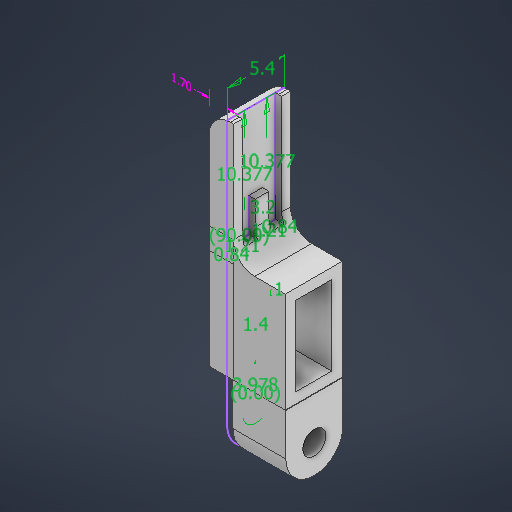
# Autodesk Inventor part: StereotaxBotHolderPartA_CH_v3
Saved by Autodesk Inventor 2026.1 (Build 301233000, 233)
## iProperties
Created: 2025-07-30
Part Number: StereotaxBotHolderPartA_CH_v3
Material: Generic
Document SubType Name: Modeling
Designer: Chris
Density: 1 g/cm^3
Appearance: Default
Author: Chris
Autodesk Inventor part; units mm, degrees
ref_plane "YZ Plane" through (0, 0, 0) normal (1, 0, 0) x (0, 1, 0)
ref_plane "XZ Plane" through (0, 0, 0) normal (0, 1, 0) x (-1, 0, 0)
ref_plane "XY Plane" through (0, 0, 0) normal (0, 0, 1) x (1, 0, 0)
sketch "Sketch1" plane through (0, 0, 0) normal (1, 0, 0) x (0, 1, 0)
  circle A0 centre (-13.4667, -0.1234) radius 1.1
  arc A1 (-13.4669, 2.577) -> (-13.4667, -2.8238) centre (-13.4667, -0.1234) ccw
  line L0 (-13.4669, 2.577) -> (-9.4882, 2.5774)
  line L1 (-9.4879, -2.8234) -> (-13.4667, -2.8238)
  line L2 (0.0118, -2.8234) -> (-9.4879, -2.8234)
  line L3 (-0.9882, -1.8234) -> (-8.4882, -1.8234)
  line L4 (-8.4882, -1.8234) -> (-8.4882, 1.5766)
  line L5 (-8.4882, 1.5766) -> (-0.9882, 1.5766)
  line L6 (-0.9882, 1.5766) -> (-0.9882, -1.8234)
  circle A2 centre (-4.7382, -0.1234) radius 1.1
  line L7 (-9.4882, 2.5774) -> (0.0115, 2.5783)
  line L8 (0.0118, -2.8234) -> (2.0118, -2.8234)
  line L9 (2.0118, 2.5766) -> (0.0115, 2.5783)
  line L10 (2.0118, 2.5766) -> (11.4892, 2.5766)
  line L11 (11.4892, -2.8234) -> (2.0118, -2.8234)
  line L12 (11.4892, -2.8234) -> (11.4892, 2.5766)
  line L13 (11.4892, 2.5766) -> (1.1118, 2.5766)
  line L14 (1.1118, 2.5766) -> (1.1118, 1.7366)
  line L15 (1.1118, 1.7366) -> (11.4892, 1.7366)
  line L16 (11.4892, 1.7366) -> (11.4892, 2.5766)
  line L17 (11.4892, -2.8234) -> (1.1118, -2.8234)
  line L18 (1.1118, -2.8234) -> (1.1118, -1.9834)
  line L19 (1.1118, -1.9834) -> (11.4892, -1.9834)
  line L20 (11.4892, -1.9834) -> (11.4892, -2.8234)
  line L21 (1.1118, -1.9834) -> (1.1118, -0.7734)
  line L22 (1.1118, 1.7366) -> (1.1118, 0.5266)
  line L23 (1.1118, 1.7366) -> (2.3218, 1.7366) construction
  line L24 (1.1118, 0.5266) -> (4.3118, 0.5266)
  line L25 (4.3118, 0.5266) -> (4.3118, -0.7734)
  line L26 (4.3118, -0.7734) -> (1.1118, -0.7734)
  line L27 (-13.4667, -0.1234) -> (-9.4882, -0.1234)
  line L28 (-13.4667, -0.1234) -> (-9.4882, -0.1234) construction
  line L29 (-9.4882, -0.1234) -> (-9.4879, -2.8234)
  line L30 (-9.4882, 2.5774) -> (-9.4882, -0.1234)
  line L31 (-9.4882, -2.8234) -> (0.0118, -2.8234)
  line L32 (0.0118, -2.8234) -> (0.0118, 2.5766)
  line L33 (0.0118, 2.5766) -> (-9.4882, 2.5766)
  line L34 (-9.4882, 2.5766) -> (-9.4882, -2.8234)
  circle A3 centre (-4.7382, -0.1234) radius 2.5
  point P0 (0, 0)
  point P1 (-9.4882, 2.5766)
  dimension "d2" = 5.4
  dimension "d3" = 10.3774
  dimension "d4" = 0.84
  dimension "d5" = 10.3774
  dimension "d6" = 0.84
  dimension "d7" = 1.21
  dimension "d8" = 1.21
  dimension "d9" = 90
  dimension "d10" = 3.2
  dimension "d11" = 3.9785
  dimension "d12" = 0
  dimension "d17" = 1
  dimension "d27" = 1.4
  constraints: 70 end point, 6 horizontal, 5 parallel, 5 perpendicular, 4 centre point, 2 equal length, 2 point on circle, 2 vertical, 3 other
  measures "d2" distance of L11.start L10.end
  measures "d3" distance of L15.end L14.end
  measures "d4" distance of L14.end L13.end
  measures "d5" distance of L18.end L19.end
  measures "d6" distance of L17.end L18.end
  measures "d7" distance of L18.end L21.end
  measures "d8" distance of L14.end L22.end
  measures "d9" angle of L22 L23
  measures "d10" distance of L25.end L26.end
  measures "d11" distance of L27.start L27.end
  measures "d12" distance between parallel lines of L27 L28
  measures "d17" distance between parallel lines of L3 L31
  measures "d27" radial gap between concentric circles of A2 A3
extrude "Extrusion1" add sketch "Sketch1" against normal blind 1.7 contours L7 L32 L2 L29 L30 | L9 L14 L22 L24 L25 L26 L21 L18 L8 L32 | L9 L10 L12 L15 L14 | L18 L19 L12 L11 L8 | L15 L12 L19 L21 L26 L25 L24 L22 | L3 A3 L5 L6 | A3 L3 | L3 A3 L5 | L3 L4 L5 A3 | L5 A3
extrude "Extrusion2" add sketch "Sketch1" along normal blind 5.5 contours L0 L30 L29 L1 A1 | L7 L32 L2 L29 L30 | A3 L3 | L5 A3
extrude "Extrusion3" cut sketch "Sketch1" against normal blind 0.05 contours L3 A3 L5 L6 | L3 A3 L5 | L3 L4 L5 A3
extrude "Extrusion5" cut sketch "Sketch1" along normal blind 0.55 contours L0 L30 L29 L1 A1
sketch "Sketch2" plane through (-1.7, 0, 0) normal (-1, 0, 0) x (0, 0, 1)
  circle A0 centre (-0.1234, -4.7382) radius 2.5 projected
  line L0 (-2.8234, 11.4892) -> (-2.8234, -9.4879) projected
  line L1 (-2.8234, -9.4879) -> (-0.1234, -9.4882) projected
  line L2 (-0.1234, -9.4882) -> (2.5774, -9.4882) projected
  line L3 (2.5774, -9.4882) -> (2.5783, 0.0115) projected
  line L4 (2.5783, 0.0115) -> (2.5766, 2.0118) projected
  line L5 (2.5766, 2.0118) -> (2.5766, 11.4892) projected
  line L6 (2.5766, 11.4892) -> (-2.8234, 11.4892) projected
  circle A1 centre (-0.1234, -4.7382) radius 1.1 projected
  point P0 (0, 0)
extrude "Extrusion6" cut sketch "Sketch2" against normal blind 0.8 contours A0
extrude "Extrusion7" add sketch "Sketch1" along normal blind 0.6 contours L9 L14 L22 L24 L25 L26 L21 L18 L8 L32 | L9 L10 L12 L15 L14 | L18 L19 L12 L11 L8
sketch "Sketch3" plane through (5.5, 0, 0) normal (1, 0, 0) x (0, 0, -1)
  line L0 (2.8234, -9.4882) -> (-2.5774, -9.4882) projected
  line L1 (-2.5766, 0.0118) -> (-2.5766, -9.4882) projected
  line L2 (-2.5766, -9.4882) -> (-2.5774, -9.4882) projected
  line L3 (-2.5774, -9.4882) -> (-2.577, -13.4669) projected
  arc A0 (-2.577, -13.4669) -> (2.8238, -13.4667) centre (0.1234, -13.4667) ccw projected
  line L4 (2.8238, -13.4667) -> (2.8234, -9.4879) projected
  line L5 (2.8234, -9.4879) -> (2.8234, 0.0118) projected
  line L6 (2.8234, 0.0118) -> (-2.5766, 0.0118) projected
  line L7 (1.8234, -0.9882) -> (1.8234, -8.4882) projected
  line L8 (1.8234, -8.4882) -> (-1.5766, -8.4882) projected
  line L9 (-1.5766, -8.4882) -> (-1.5766, -0.9882) projected
  line L10 (-1.5766, -0.9882) -> (1.8234, -0.9882) projected
  circle A1 centre (0.1234, -13.4667) radius 1.1 projected
  point P0 (0, 0)
extrude "Extrusion8" add sketch "Sketch3" along normal blind 0.05 contours L4 A0 L3 L0
fillet "Fillet1" radius 2 2 edges at (0.6, 0.0117, -0.1234) (-1.7, 11.4892, -0.1234)
body "Solid1"
